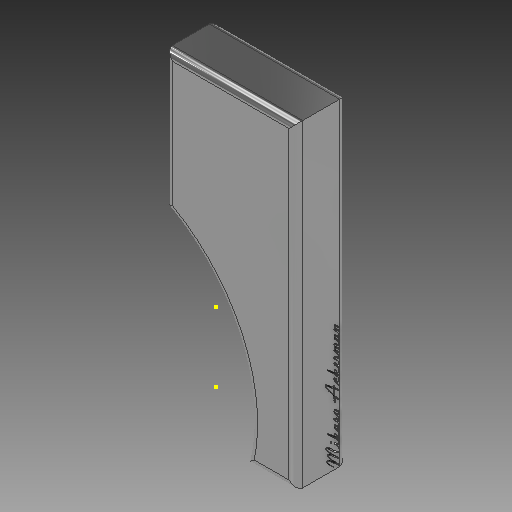
# Autodesk Inventor part: Wire Attachement
Saved by Autodesk Inventor 2021 (Build 250183000, 183)
## iProperties
Created: 2021-05-04
Part Number: Wire Attachement
Material: Generic
Document SubType Name: Modeling
Designer: AHUJA
Density: 1 g/cm^3
Appearance: Default
Author: AHUJA
Autodesk Inventor part; units mm, degrees
ref_plane "YZ Plane" through (0, 0, 0) normal (1, 0, 0) x (0, 1, 0)
ref_plane "XZ Plane" through (0, 0, 0) normal (0, 1, 0) x (-1, 0, 0)
ref_plane "XY Plane" through (0, 0, 0) normal (0, 0, 1) x (1, 0, 0)
sketch "Sketch1" plane through (0, 0, 0) normal (0, 0, 1) x (1, 0, 0)
  line L0 (0, 0) -> (18.946, 0)
  line L1 (18.946, 0) -> (18.946, 46.274)
  line L2 (18.946, 46.274) -> (0, 46.274)
  line L3 (0, 46.274) -> (0, 0)
  line L4 (0, 46.274) -> (0, 26.493)
  line L5 (18.946, 0) -> (11.661, 0)
  arc A0 (11.661, 0) -> (0, 26.493) centre (-11.0706, 5.8074) ccw
  dimension "d0" = 46.274
  dimension "d1" = 18.946
  dimension "d2" = 19.781
  dimension "d3" = 7.285
  constraints: 12 end point, 2 parallel, 2 point on circle, 2 point on line, 1 centre point, 1 horizontal, 1 perpendicular
  measures "d0" distance of L0.end L1.end
  measures "d1" distance of L1.end L2.end
  measures "d2" distance of L2.end L4.end
  measures "d3" distance of L0.end L5.end
extrude "Extrusion1" add sketch "Sketch1" along normal blind 7.366 contours A0 L3 L2 L1 L0
fillet "Fillet1" radius 1 10 edges at (10.403, 15.2591, 7.366) (0, 36.3835, 7.366) (9.473, 46.274, 7.366) (18.946, 23.137, 7.366) (15.3035, 0, 7.366) (18.946, 23.137, 0) (15.3035, 0, 0) (10.403, 15.2591, 0) (0, 36.3835, 0) (9.473, 46.274, 0)
sketch "Sketch2" plane through (11.661, 0, 1) normal (0, -1, 0) x (1, 0, 0)
  point P0 (-11.661, -1)
sketch "Sketch3" plane through (11.661, 0, 1) normal (0, -1, 0) x (1, 0, 0)
  line L0 (1.21, 5.156) -> (6.075, 5.156)
  line L1 (6.075, 5.156) -> (6.075, 0.21)
  line L2 (6.075, 0.21) -> (1.21, 0.21)
  line L3 (1.21, 0.21) -> (1.21, 5.156)
  line L4 (6.285, 6.366) -> (1.2531, 6.366) projected
  line L5 (1.2531, -1) -> (6.285, -1) projected
  line L6 (7.285, 0) -> (7.285, 5.366) projected
  line L7 (0, 0) -> (0, 5.366) projected
  point P0 (-11.661, -1)
  dimension "d7" = 1.21
  dimension "d8" = 1.21
  dimension "d9" = 1.21
  dimension "d10" = 1.21
  constraints: 8 end point, 2 parallel, 1 horizontal, 1 perpendicular
  measures "d7" distance between parallel lines of L4 L0
  measures "d8" distance between parallel lines of L5 L2
  measures "d9" distance between parallel lines of L6 L1
  measures "d10" distance between parallel lines of L7 L3
extrude "Extrusion2" cut sketch "Sketch3" against normal blind 10.16
fillet "Fillet2" radius 0.25 4 edges at (12.871, 5.08, 1.21) (12.871, 5.08, 6.156) (17.736, 5.08, 1.21) (17.736, 5.08, 6.156)
sketch "Sketch4" plane through (11.661, 10.16, 1) normal (0, -1, 0) x (1, 0, 0)
  line L0 (1.61, 3.51) -> (2.41, 3.51)
  line L1 (2.41, 3.51) -> (2.41, 2.41)
  line L2 (2.41, 2.41) -> (1.61, 2.41)
  line L3 (1.61, 2.41) -> (1.61, 3.51)
  line L4 (1.21, 0.46) -> (1.21, 4.906) projected
  line L5 (5.825, 0.21) -> (1.46, 0.21) projected
  line L6 (2.81, 3.51) -> (3.61, 3.51)
  line L7 (3.61, 3.51) -> (3.61, 2.41)
  line L8 (3.61, 2.41) -> (2.81, 2.41)
  line L9 (2.81, 2.41) -> (2.81, 3.51)
  point P0 (-11.661, -1)
  dimension "d14" = 0.4
  dimension "d15" = 0.8
  dimension "d16" = 1.1
  dimension "d17" = 2.2
  dimension "d18" = 0.8
  dimension "d19" = 1.1
  dimension "d20" = 0.4
  dimension "d21" = 2.2
  constraints: 16 end point, 4 parallel, 2 horizontal, 2 perpendicular
  measures "d14" distance between parallel lines of L4 L3
  measures "d15" distance of L0.start L0.end
  measures "d16" distance of L0.end L1.end
  measures "d17" distance between parallel lines of L5 L2
  measures "d18" distance of L6.start L6.end
  measures "d19" distance of L6.end L7.end
  measures "d20" distance between parallel lines of L1 L9
  measures "d21" distance between parallel lines of L5 L8
extrude "Extrusion3" add sketch "Sketch4" along normal blind 10.16
fillet "Fillet3" radius 0.15 8 edges at (15.271, 5.08, 4.51) (15.271, 5.08, 3.41) (14.071, 5.08, 3.41) (14.071, 5.08, 4.51) (14.471, 5.08, 4.51) (14.471, 5.08, 3.41) (13.271, 5.08, 4.51) (13.271, 5.08, 3.41)
sketch "Sketch5" plane through (11.661, 10.16, 1) normal (0, -1, 0) x (1, 0, 0)
  point P0 (-11.661, -1)
sketch "Sketch6" plane through (11.661, 10.16, 1) normal (0, -1, 0) x (1, 0, 0)
  line L0 (3.91, 3.91) -> (5.91, 3.91)
  line L1 (5.91, 3.91) -> (5.91, 2.21)
  line L2 (5.91, 2.21) -> (3.91, 2.21)
  line L3 (3.91, 2.21) -> (3.91, 3.91)
  line L4 (1.46, 5.156) -> (5.825, 5.156) projected
  line L5 (5.825, 0.21) -> (1.46, 0.21) projected
  line L6 (3.61, 2.56) -> (3.61, 3.36) projected
  point P0 (-11.661, -1)
  dimension "d25" = 2
  dimension "d26" = 1.7
  dimension "d28" = 2
  dimension "d29" = 0.3
  constraints: 8 end point, 2 parallel, 1 horizontal, 1 perpendicular
  measures "d25" distance of L0.start L0.end
  measures "d26" distance of L2.end L0.start
  measures "d28" distance between parallel lines of L5 L2
  measures "d29" distance between parallel lines of L6 L3
extrude "Extrusion4" add sketch "Sketch6" along normal blind 10.16
sketch "Sketch7" plane through (11.661, 0, 1) normal (0, -1, 0) x (1, 0, 0)
  line L0 (4.31, 3.51) -> (5.51, 3.51)
  line L1 (5.51, 3.51) -> (5.51, 2.61)
  line L2 (5.51, 2.61) -> (4.31, 2.61)
  line L3 (4.31, 2.61) -> (4.31, 3.51)
  line L4 (5.91, 3.91) -> (3.91, 3.91) projected
  line L5 (3.91, 2.21) -> (5.91, 2.21) projected
  line L6 (5.91, 2.21) -> (5.91, 3.91) projected
  line L7 (3.91, 3.91) -> (3.91, 2.21) projected
  point P0 (-11.661, -1)
  dimension "d32" = 0.4
  dimension "d33" = 0.4
  dimension "d34" = 0.4
  dimension "d35" = 0.4
  constraints: 8 end point, 2 parallel, 1 horizontal, 1 perpendicular
  measures "d32" distance between parallel lines of L4 L0
  measures "d33" distance between parallel lines of L5 L2
  measures "d34" distance between parallel lines of L6 L1
  measures "d35" distance between parallel lines of L3 L7
extrude "Extrusion5" cut sketch "Sketch7" against normal blind 10.16 contours L0 L1 L2 L3
fillet "Fillet4" radius 0.15 4 edges at (17.571, 5.08, 4.91) (17.571, 5.08, 3.21) (15.571, 5.08, 4.91) (15.571, 5.08, 3.21)
sketch "Sketch8" plane through (18.946, 0, 1) normal (1, 0, 0) x (0, 0, -1)
  line L0 (-2.1201, 0.0445) -> (-2.1201, 18.5514) construction
  line L1 (-2.1201, 18.5514) -> (-0.0042, 18.5514) construction
  line L2 (-0.0042, 18.5514) -> (-0.0042, 0.0445) construction
  line L3 (-0.0042, 0.0445) -> (-2.1201, 0.0445) construction
  spline S0 degree 2 poles (-1.0025, 1.9649) (-2.0042, 2.9545) (-2.0042, 3.2314) knots 0 0 0 1 1 1
  spline S1 degree 2 poles (-2.0042, 3.2314) (-2.0042, 3.3473) (-1.8952, 3.3473) knots 0 0 0 1 1 1
  spline S2 degree 2 poles (-1.8952, 3.3473) (-1.7932, 3.3473) (-1.6686, 3.2642) knots 0 0 0 1 1 1
  spline S3 degree 2 poles (-1.6686, 3.2642) (-1.5804, 3.202) (-0.8624, 2.5168) knots 0 0 0 1 1 1
  spline S4 degree 2 poles (-0.8624, 2.5168) (-0.2291, 1.9459) (-0.1184, 1.9459) knots 0 0 0 1 1 1
  spline S5 degree 2 poles (-0.1184, 1.9459) (-0.0804, 1.9459) (-0.0717, 2.0566) (-0.0596, 2.0566) knots 0 0 0 1 2 2 2
  spline S6 degree 2 poles (-0.0596, 2.0566) (-0.0198, 2.0566) (-0.0198, 1.9701) knots 0 0 0 1 1 1
  spline S7 degree 2 poles (-0.0198, 1.9701) (-0.0198, 1.8473) (-0.1357, 1.8473) knots 0 0 0 1 1 1
  spline S8 degree 2 poles (-0.1357, 1.8473) (-0.3502, 1.8473) (-0.9437, 2.3802) knots 0 0 0 1 1 1
  spline S9 degree 2 poles (-0.9437, 2.3802) (-1.153, 2.567) (-1.6755, 3.0878) knots 0 0 0 1 1 1
  spline S10 degree 2 poles (-1.6755, 3.0878) (-1.852, 3.266) (-1.9229, 3.266) knots 0 0 0 1 1 1
  spline S11 degree 2 poles (-1.9229, 3.266) (-1.9506, 3.266) (-1.9506, 3.2383) knots 0 0 0 1 1 1
  spline S12 degree 2 poles (-1.9506, 3.2383) (-1.9506, 3.1397) (-1.5717, 2.6829) knots 0 0 0 1 1 1
  spline S13 degree 2 poles (-1.5717, 2.6829) (-1.2672, 2.3179) (-1.0873, 2.1379) knots 0 0 0 1 1 1
  spline S14 degree 2 poles (-1.0873, 2.1379) (-0.9143, 1.9649) (-0.5994, 1.6829) knots 0 0 0 1 1 1
  spline S15 degree 2 poles (-0.5994, 1.6829) (-0.0302, 1.176) (-0.0302, 1.1604) knots 0 0 0 1 1 1
  spline S16 degree 2 poles (-0.0302, 1.1604) (-0.0302, 1.1397) (-0.0838, 1.0808) (-0.1063, 1.0808) knots 0 0 0 1 2 2 2
  spline S17 degree 2 poles (-0.1063, 1.0808) (-0.1617, 1.0808) (-1.5942, 2.2936) (-1.7084, 2.2936) knots 0 0 0 1 2 2 2
  spline S18 degree 2 poles (-1.7084, 2.2936) (-1.7378, 2.2936) (-1.7378, 2.266) knots 0 0 0 1 1 1
  spline S19 degree 2 poles (-1.7378, 2.266) (-1.7378, 2.1916) (-1.5094, 1.8888) knots 0 0 0 1 1 1
  spline S20 degree 2 poles (-1.5094, 1.8888) (-1.2983, 1.6085) (-0.9783, 1.2729) knots 0 0 0 1 1 1
  line L4 (-0.9783, 1.2729) -> (-0.4056, 0.695)
  line L5 (-0.4056, 0.695) -> (-0.1876, 0.4926)
  spline S21 degree 2 poles (-0.1876, 0.4926) (-0.0042, 0.3231) (-0.0042, 0.3092) knots 0 0 0 1 1 1
  spline S22 degree 2 poles (-0.0042, 0.3092) (-0.0042, 0.2867) (-0.0267, 0.2521) knots 0 0 0 1 1 1
  spline S23 degree 2 poles (-0.0267, 0.2521) (-0.0509, 0.2141) (-0.0734, 0.2141) knots 0 0 0 1 1 1
  spline S24 degree 2 poles (-0.0734, 0.2141) (-0.1201, 0.2141) (-0.5215, 0.5722) knots 0 0 0 1 1 1
  line L6 (-0.5215, 0.5722) -> (-1.2724, 1.24)
  spline S25 degree 2 poles (-1.2724, 1.24) (-1.6945, 1.5999) (-1.7949, 1.5999) knots 0 0 0 1 1 1
  spline S26 degree 2 poles (-1.7949, 1.5999) (-1.8312, 1.5999) (-1.8312, 1.5635) knots 0 0 0 1 1 1
  spline S27 degree 2 poles (-1.8312, 1.5635) (-1.8312, 1.4597) (-1.5665, 1.1345) knots 0 0 0 1 1 1
  spline S28 degree 2 poles (-1.5665, 1.1345) (-1.3693, 0.8905) (-0.8676, 0.439) knots 0 0 0 1 1 1
  spline S29 degree 2 poles (-0.8676, 0.439) (-0.8364, 0.4096) (-0.8364, 0.3923) knots 0 0 0 1 1 1
  spline S30 degree 2 poles (-0.8364, 0.3923) (-0.8364, 0.3611) (-0.8606, 0.3611) knots 0 0 0 1 1 1
  spline S31 degree 2 poles (-0.8606, 0.3611) (-0.897, 0.3611) (-1.1842, 0.6103) knots 0 0 0 1 1 1
  spline S32 degree 2 poles (-1.1842, 0.6103) (-1.3866, 0.7902) (-1.6132, 1.0618) knots 0 0 0 1 1 1
  spline S33 degree 2 poles (-1.6132, 1.0618) (-1.9039, 1.4148) (-1.9039, 1.5722) knots 0 0 0 1 1 1
  spline S34 degree 2 poles (-1.9039, 1.5722) (-1.9039, 1.6777) (-1.788, 1.6777) knots 0 0 0 1 1 1
  spline S35 degree 2 poles (-1.788, 1.6777) (-1.5942, 1.6777) (-0.9662, 1.1639) knots 0 0 0 1 1 1
  spline S36 degree 2 poles (-0.9662, 1.1639) (-1.8018, 2.0411) (-1.8018, 2.266) knots 0 0 0 1 1 1
  spline S37 degree 2 poles (-1.8018, 2.266) (-1.8018, 2.3715) (-1.6928, 2.3715) knots 0 0 0 1 1 1
  spline S38 degree 2 poles (-1.6928, 2.3715) (-1.5215, 2.3715) (-1.0025, 1.9649) knots 0 0 0 1 1 1
  spline S39 degree 2 poles (-0.1167, 2.9459) (-0.0786, 2.9459) (-0.0786, 3.0289) knots 0 0 0 1 1 1
  spline S40 degree 2 poles (-0.0786, 3.0289) (-0.0786, 3.048) (-0.0544, 3.048) knots 0 0 0 1 1 1
  spline S41 degree 2 poles (-0.0544, 3.048) (-0.0267, 3.048) (-0.0267, 2.9528) knots 0 0 0 1 1 1
  spline S42 degree 2 poles (-0.0267, 2.9528) (-0.0267, 2.8455) (-0.1288, 2.8455) knots 0 0 0 1 1 1
  spline S43 degree 2 poles (-0.1288, 2.8455) (-0.2499, 2.8455) (-0.6305, 3.1639) knots 0 0 0 1 1 1
  line L7 (-0.6305, 3.1639) -> (-0.3122, 2.7746)
  spline S44 degree 2 poles (-0.3122, 2.7746) (-0.0302, 2.4286) (-0.0302, 2.2729) knots 0 0 0 1 1 1
  spline S45 degree 2 poles (-0.0302, 2.2729) (-0.0302, 2.2556) (-0.0492, 2.2556) knots 0 0 0 1 1 1
  spline S46 degree 2 poles (-0.0492, 2.2556) (-0.0769, 2.2556) (-0.0821, 2.285) knots 0 0 0 1 1 1
  spline S47 degree 2 poles (-0.0821, 2.285) (-0.0994, 2.3732) (-0.1409, 2.4476) knots 0 0 0 1 1 1
  spline S48 degree 2 poles (-0.1409, 2.4476) (-0.1911, 2.5411) (-0.4298, 2.8421) knots 0 0 0 1 1 1
  line L8 (-0.4298, 2.8421) -> (-0.7949, 3.2781)
  spline S49 degree 2 poles (-0.7949, 3.2781) (-0.8053, 3.3075) (-0.8053, 3.3559) knots 0 0 0 1 1 1
  spline S50 degree 2 poles (-0.8053, 3.3559) (-0.8053, 3.4044) (-0.7499, 3.4044) knots 0 0 0 1 1 1
  spline S51 degree 2 poles (-0.7499, 3.4044) (-0.6893, 3.4044) (-0.1634, 2.9459) (-0.1167, 2.9459) knots 0 0 0 1 2 2 2
  spline S52 degree 2 poles (-1.1046, 3.5757) (-1.1046, 3.5064) (-1.1738, 3.5064) knots 0 0 0 1 1 1
  spline S53 degree 2 poles (-1.1738, 3.5064) (-1.2326, 3.5064) (-1.2793, 3.5757) knots 0 0 0 1 1 1
  spline S54 degree 2 poles (-1.2793, 3.5757) (-1.3226, 3.6397) (-1.3226, 3.702) knots 0 0 0 1 1 1
  spline S55 degree 2 poles (-1.3226, 3.702) (-1.3226, 3.7763) (-1.2413, 3.7763) knots 0 0 0 1 1 1
  spline S56 degree 2 poles (-1.2413, 3.7763) (-1.1824, 3.7763) (-1.1409, 3.702) knots 0 0 0 1 1 1
  spline S57 degree 2 poles (-1.1409, 3.702) (-1.1046, 3.6379) (-1.1046, 3.5757) knots 0 0 0 1 1 1
  line L9 (-0.6893, 3.977) -> (-0.3676, 3.5947)
  line L10 (-0.3676, 3.5947) -> (-0.1617, 3.3317)
  spline S58 degree 2 poles (-0.1617, 3.3317) (-0.0302, 3.1449) (-0.0302, 3.0255) knots 0 0 0 1 1 1
  spline S59 degree 2 poles (-0.0302, 3.0255) (-0.0302, 3.0082) (-0.0492, 3.0082) knots 0 0 0 1 1 1
  spline S60 degree 2 poles (-0.0492, 3.0082) (-0.0752, 3.0082) (-0.0821, 3.0376) knots 0 0 0 1 1 1
  spline S61 degree 2 poles (-0.0821, 3.0376) (-0.1271, 3.2244) (-0.3935, 3.5462) knots 0 0 0 1 1 1
  line L11 (-0.3935, 3.5462) -> (-0.7326, 3.9528)
  spline S62 degree 2 poles (-0.7326, 3.9528) (-0.8502, 4.093) (-1.1963, 4.4044) knots 0 0 0 1 1 1
  line L12 (-1.1963, 4.4044) -> (-1.653, 4.804)
  spline S63 degree 2 poles (-1.653, 4.804) (-1.7655, 4.8992) (-1.7655, 4.9372) knots 0 0 0 1 1 1
  spline S64 degree 2 poles (-1.7655, 4.9372) (-1.7655, 4.9874) (-1.7153, 4.9874) knots 0 0 0 1 1 1
  spline S65 degree 2 poles (-1.7153, 4.9874) (-1.653, 4.9874) (-1.5008, 4.8646) knots 0 0 0 1 1 1
  line L13 (-1.5008, 4.8646) -> (-1.3001, 4.6881)
  line L14 (-1.3001, 4.6881) -> (-0.6444, 4.1189)
  spline S66 degree 2 poles (-0.6444, 4.1189) (-0.7949, 4.3282) (-0.7949, 4.4269) knots 0 0 0 1 1 1
  spline S67 degree 2 poles (-0.7949, 4.4269) (-0.7949, 4.5428) (-0.6807, 4.5428) knots 0 0 0 1 1 1
  spline S68 degree 2 poles (-0.6807, 4.5428) (-0.5527, 4.5428) (-0.461, 4.3179) knots 0 0 0 1 1 1
  spline S69 degree 2 poles (-0.461, 4.3179) (-0.3866, 4.1345) (-0.3849, 3.977) knots 0 0 0 1 1 1
  spline S70 degree 2 poles (-0.3849, 3.977) (-0.2637, 4.0272) (-0.1098, 4.1085) knots 0 0 0 1 1 1
  spline S71 degree 2 poles (-0.1098, 4.1085) (-0.0769, 4.1362) (-0.0769, 4.1968) knots 0 0 0 1 1 1
  spline S72 degree 2 poles (-0.0769, 4.1968) (-0.0769, 4.2175) (-0.0544, 4.2175) knots 0 0 0 1 1 1
  spline S73 degree 2 poles (-0.0544, 4.2175) (-0.0233, 4.2175) (-0.0233, 4.1068) knots 0 0 0 1 1 1
  spline S74 degree 2 poles (-0.0233, 4.1068) (-0.0233, 4.0514) (-0.0509, 4.0134) knots 0 0 0 1 1 1
  spline S75 degree 2 poles (-0.0509, 4.0134) (-0.0752, 3.9788) (-0.3329, 3.8577) knots 0 0 0 1 1 1
  line L15 (-0.3329, 3.8577) -> (-0.1617, 3.7141)
  spline S76 degree 2 poles (-0.1617, 3.7141) (-0.0215, 3.5947) (-0.0215, 3.5705) knots 0 0 0 1 1 1
  spline S77 degree 2 poles (-0.0215, 3.5705) (-0.0215, 3.5099) (-0.0925, 3.5099) knots 0 0 0 1 1 1
  spline S78 degree 2 poles (-0.0925, 3.5099) (-0.134, 3.5099) (-0.4056, 3.7348) knots 0 0 0 1 1 1
  line L16 (-0.4056, 3.7348) -> (-0.6893, 3.977)
  spline S79 degree 2 poles (-0.4177, 3.9338) (-0.4454, 4.1466) (-0.6253, 4.4234) (-0.6893, 4.4234) knots 0 0 0 1 2 2 2
  spline S80 degree 2 poles (-0.6893, 4.4234) (-0.7222, 4.4234) (-0.7222, 4.3819) knots 0 0 0 1 1 1
  spline S81 degree 2 poles (-0.7222, 4.3819) (-0.7222, 4.2262) (-0.4177, 3.9338) knots 0 0 0 1 1 1
  spline S82 degree 2 poles (-0.3312, 4.721) (-0.0302, 4.3386) (-0.0302, 4.195) knots 0 0 0 1 1 1
  spline S83 degree 2 poles (-0.0302, 4.195) (-0.0302, 4.1777) (-0.0492, 4.1777) knots 0 0 0 1 1 1
  spline S84 degree 2 poles (-0.0492, 4.1777) (-0.0769, 4.1777) (-0.0821, 4.2123) knots 0 0 0 1 1 1
  spline S85 degree 2 poles (-0.0821, 4.2123) (-0.1028, 4.3455) (-0.2897, 4.5843) knots 0 0 0 1 1 1
  line L17 (-0.2897, 4.5843) -> (-0.4333, 4.7677)
  line L18 (-0.4333, 4.7677) -> (-0.6686, 5.0635)
  spline S86 degree 2 poles (-0.6686, 5.0635) (-0.8087, 5.266) (-0.8087, 5.4113) knots 0 0 0 1 1 1
  spline S87 degree 2 poles (-0.8087, 5.4113) (-0.8087, 5.5186) (-0.7015, 5.5307) knots 0 0 0 1 1 1
  spline S88 degree 2 poles (-0.7015, 5.5307) (-0.7551, 5.586) (-0.7551, 5.6085) knots 0 0 0 1 1 1
  spline S89 degree 2 poles (-0.7551, 5.6085) (-0.7551, 5.6552) (-0.7153, 5.6552) knots 0 0 0 1 1 1
  spline S90 degree 2 poles (-0.7153, 5.6552) (-0.6651, 5.6552) (-0.1547, 5.2175) (-0.1115, 5.2175) knots 0 0 0 1 2 2 2
  spline S91 degree 2 poles (-0.1115, 5.2175) (-0.0821, 5.2175) (-0.0786, 5.3092) (-0.0561, 5.3092) knots 0 0 0 1 2 2 2
  spline S92 degree 2 poles (-0.0561, 5.3092) (-0.0267, 5.3092) (-0.0267, 5.2141) knots 0 0 0 1 1 1
  spline S93 degree 2 poles (-0.0267, 5.2141) (-0.0267, 5.1189) (-0.1115, 5.1189) knots 0 0 0 1 1 1
  spline S94 degree 2 poles (-0.1115, 5.1189) (-0.179, 5.1189) (-0.3018, 5.195) knots 0 0 0 1 1 1
  line L19 (-0.3018, 5.195) -> (-0.1513, 5.0186)
  spline S95 degree 2 poles (-0.1513, 5.0186) (-0.0544, 4.8888) (-0.0544, 4.8109) knots 0 0 0 1 1 1
  spline S96 degree 2 poles (-0.0544, 4.8109) (-0.0544, 4.6881) (-0.179, 4.6881) knots 0 0 0 1 1 1
  spline S97 degree 2 poles (-0.179, 4.6881) (-0.2482, 4.6881) (-0.3312, 4.721) knots 0 0 0 1 1 1
  spline S98 degree 2 poles (-0.7499, 5.4303) (-0.7499, 5.3455) (-0.2464, 4.8179) (-0.1617, 4.8179) knots 0 0 0 1 2 2 2
  spline S99 degree 2 poles (-0.1617, 4.8179) (-0.1236, 4.8179) (-0.1236, 4.8542) knots 0 0 0 1 1 1
  spline S100 degree 2 poles (-0.1236, 4.8542) (-0.1236, 4.9372) (-0.6167, 5.4718) (-0.7032, 5.4718) knots 0 0 0 1 2 2 2
  spline S101 degree 2 poles (-0.7032, 5.4718) (-0.7499, 5.4718) (-0.7499, 5.4303) knots 0 0 0 1 1 1
  spline S102 degree 2 poles (-0.2741, 5.7383) (-0.0302, 5.4407) (-0.0302, 5.2867) knots 0 0 0 1 1 1
  spline S103 degree 2 poles (-0.0302, 5.2867) (-0.0302, 5.2694) (-0.0475, 5.2694) knots 0 0 0 1 1 1
  spline S104 degree 2 poles (-0.0475, 5.2694) (-0.0752, 5.2694) (-0.0821, 5.2988) knots 0 0 0 1 1 1
  spline S105 degree 2 poles (-0.0821, 5.2988) (-0.0942, 5.3507) (-0.1392, 5.4615) knots 0 0 0 1 1 1
  spline S106 degree 2 poles (-0.1392, 5.4615) (-0.1945, 5.5635) (-0.544, 5.984) knots 0 0 0 1 1 1
  spline S107 degree 2 poles (-0.544, 5.984) (-0.8745, 6.3819) (-0.8745, 6.3923) knots 0 0 0 1 1 1
  spline S108 degree 2 poles (-0.8745, 6.3923) (-0.8745, 6.4251) (-0.8174, 6.4891) (-0.7845, 6.4891) knots 0 0 0 1 2 2 2
  spline S109 degree 2 poles (-0.7845, 6.4891) (-0.6807, 6.4891) (-0.4177, 6.3265) knots 0 0 0 1 1 1
  spline S110 degree 2 poles (-0.4177, 6.3265) (-0.1911, 6.1847) (-0.0786, 6.0791) knots 0 0 0 1 1 1
  spline S111 degree 2 poles (-0.0786, 6.0791) (-0.0786, 6.1414) (-0.0561, 6.1414) knots 0 0 0 1 1 1
  spline S112 degree 2 poles (-0.0561, 6.1414) (-0.0267, 6.1414) (-0.0267, 6.0808) knots 0 0 0 1 1 1
  spline S113 degree 2 poles (-0.0267, 6.0808) (-0.0267, 6.0653) (-0.0371, 6.0047) (-0.0371, 5.9874) knots 0 0 0 1 2 2 2
  spline S114 degree 2 poles (-0.0371, 5.9874) (-0.0371, 5.977) (-0.0284, 5.9303) (-0.0284, 5.9199) knots 0 0 0 1 2 2 2
  spline S115 degree 2 poles (-0.0284, 5.9199) (-0.0284, 5.7383) (-0.2741, 5.7383) knots 0 0 0 1 1 1
  spline S116 degree 2 poles (-0.1478, 5.9649) (-0.2309, 6.0653) (-0.435, 6.1847) knots 0 0 0 1 1 1
  spline S117 degree 2 poles (-0.435, 6.1847) (-0.6236, 6.2954) (-0.7689, 6.3404) knots 0 0 0 1 1 1
  line L20 (-0.7689, 6.3404) -> (-0.3537, 5.83)
  spline S118 degree 2 poles (-0.3537, 5.83) (-0.3451, 5.8819) (-0.2707, 5.9182) knots 0 0 0 1 1 1
  line L21 (-0.2707, 5.9182) -> (-0.1478, 5.9649)
  line L22 (-0.1046, 5.9251) -> (-0.2188, 5.8853)
  spline S119 degree 2 poles (-0.2188, 5.8853) (-0.3018, 5.8525) (-0.3018, 5.8231) knots 0 0 0 1 1 1
  spline S120 degree 2 poles (-0.3018, 5.8231) (-0.3018, 5.7919) (-0.2534, 5.7919) knots 0 0 0 1 1 1
  spline S121 degree 2 poles (-0.2534, 5.7919) (-0.2032, 5.7919) (-0.1513, 5.8196) knots 0 0 0 1 1 1
  spline S122 degree 2 poles (-0.1513, 5.8196) (-0.0925, 5.8525) (-0.0925, 5.8975) knots 0 0 0 1 1 1
  spline S123 degree 2 poles (-0.0925, 5.8975) (-0.0925, 5.9148) (-0.1046, 5.9251) knots 0 0 0 1 1 1
  spline S124 degree 2 poles (-0.3312, 6.6449) (-0.0302, 6.2625) (-0.0302, 6.1189) knots 0 0 0 1 1 1
  spline S125 degree 2 poles (-0.0302, 6.1189) (-0.0302, 6.1016) (-0.0492, 6.1016) knots 0 0 0 1 1 1
  spline S126 degree 2 poles (-0.0492, 6.1016) (-0.0769, 6.1016) (-0.0821, 6.1362) knots 0 0 0 1 1 1
  spline S127 degree 2 poles (-0.0821, 6.1362) (-0.1028, 6.2694) (-0.2897, 6.5082) knots 0 0 0 1 1 1
  line L23 (-0.2897, 6.5082) -> (-0.4333, 6.6916)
  line L24 (-0.4333, 6.6916) -> (-0.6686, 6.9874)
  spline S128 degree 2 poles (-0.6686, 6.9874) (-0.8087, 7.1898) (-0.8087, 7.3352) knots 0 0 0 1 1 1
  spline S129 degree 2 poles (-0.8087, 7.3352) (-0.8087, 7.4424) (-0.7015, 7.4545) knots 0 0 0 1 1 1
  spline S130 degree 2 poles (-0.7015, 7.4545) (-0.7551, 7.5099) (-0.7551, 7.5324) knots 0 0 0 1 1 1
  spline S131 degree 2 poles (-0.7551, 7.5324) (-0.7551, 7.5791) (-0.7153, 7.5791) knots 0 0 0 1 1 1
  spline S132 degree 2 poles (-0.7153, 7.5791) (-0.6651, 7.5791) (-0.1547, 7.1414) (-0.1115, 7.1414) knots 0 0 0 1 2 2 2
  spline S133 degree 2 poles (-0.1115, 7.1414) (-0.0821, 7.1414) (-0.0786, 7.2331) (-0.0561, 7.2331) knots 0 0 0 1 2 2 2
  spline S134 degree 2 poles (-0.0561, 7.2331) (-0.0267, 7.2331) (-0.0267, 7.1379) knots 0 0 0 1 1 1
  spline S135 degree 2 poles (-0.0267, 7.1379) (-0.0267, 7.0428) (-0.1115, 7.0428) knots 0 0 0 1 1 1
  spline S136 degree 2 poles (-0.1115, 7.0428) (-0.179, 7.0428) (-0.3018, 7.1189) knots 0 0 0 1 1 1
  line L25 (-0.3018, 7.1189) -> (-0.1513, 6.9424)
  spline S137 degree 2 poles (-0.1513, 6.9424) (-0.0544, 6.8127) (-0.0544, 6.7348) knots 0 0 0 1 1 1
  spline S138 degree 2 poles (-0.0544, 6.7348) (-0.0544, 6.612) (-0.179, 6.612) knots 0 0 0 1 1 1
  spline S139 degree 2 poles (-0.179, 6.612) (-0.2482, 6.612) (-0.3312, 6.6449) knots 0 0 0 1 1 1
  spline S140 degree 2 poles (-0.7499, 7.3542) (-0.7499, 7.2694) (-0.2464, 6.7417) (-0.1617, 6.7417) knots 0 0 0 1 2 2 2
  spline S141 degree 2 poles (-0.1617, 6.7417) (-0.1236, 6.7417) (-0.1236, 6.7781) knots 0 0 0 1 1 1
  spline S142 degree 2 poles (-0.1236, 6.7781) (-0.1236, 6.8611) (-0.6167, 7.3957) (-0.7032, 7.3957) knots 0 0 0 1 2 2 2
  spline S143 degree 2 poles (-0.7032, 7.3957) (-0.7499, 7.3957) (-0.7499, 7.3542) knots 0 0 0 1 1 1
  line L26 (-0.8537, 10.4199) -> (-0.8537, 10.5497)
  spline S144 degree 2 poles (-0.8537, 10.5497) (-0.8433, 10.6449) (-0.7949, 10.6449) knots 0 0 0 1 1 1
  spline S145 degree 2 poles (-0.7949, 10.6449) (-0.7637, 10.6449) (-0.7637, 10.5757) knots 0 0 0 1 1 1
  line L27 (-0.7637, 10.5757) -> (-0.7689, 10.484)
  line L28 (-0.7689, 10.484) -> (-0.7672, 10.349)
  line L29 (-0.7672, 10.349) -> (-0.3987, 10.0584)
  spline S146 degree 2 poles (-0.3987, 10.0584) (-0.0302, 9.7625) (-0.0302, 9.7314) knots 0 0 0 1 1 1
  spline S147 degree 2 poles (-0.0302, 9.7314) (-0.0302, 9.7037) (-0.0717, 9.6812) knots 0 0 0 1 1 1
  spline S148 degree 2 poles (-0.0717, 9.6812) (-0.1063, 9.6587) (-0.1357, 9.6587) knots 0 0 0 1 1 1
  spline S149 degree 2 poles (-0.1357, 9.6587) (-0.1807, 9.6587) (-0.7672, 10.1449) knots 0 0 0 1 1 1
  line L30 (-0.7672, 10.1449) -> (-0.7672, 10.0341)
  spline S150 degree 2 poles (-0.7672, 10.0341) (-0.7655, 9.8006) (-0.743, 9.3404) knots 0 0 0 1 1 1
  line L31 (-0.743, 9.3404) -> (-0.3295, 8.8594)
  line L32 (-0.3295, 8.8594) -> (-0.1617, 8.6708)
  spline S151 degree 2 poles (-0.1617, 8.6708) (-0.0302, 8.5203) (-0.0302, 8.4874) knots 0 0 0 1 1 1
  spline S152 degree 2 poles (-0.0302, 8.4874) (-0.0302, 8.4476) (-0.0717, 8.4476) knots 0 0 0 1 1 1
  spline S153 degree 2 poles (-0.0717, 8.4476) (-0.1236, 8.4476) (-0.4679, 8.8594) knots 0 0 0 1 1 1
  line L33 (-0.4679, 8.8594) -> (-0.7395, 9.1864)
  spline S154 degree 2 poles (-0.7395, 9.1864) (-0.7084, 8.5324) (-0.672, 8.5116) knots 0 0 0 1 1 1
  line L34 (-0.672, 8.5116) -> (-0.6703, 8.5116)
  spline S155 degree 2 poles (-0.6703, 8.5116) (-0.6426, 8.5116) (-0.6426, 8.7158) knots 0 0 0 1 1 1
  line L35 (-0.6426, 8.7158) -> (-0.6461, 8.9061)
  spline S156 degree 2 poles (-0.6461, 8.9061) (-0.6461, 8.9442) (-0.6288, 8.9442) knots 0 0 0 1 1 1
  spline S157 degree 2 poles (-0.6288, 8.9442) (-0.589, 8.9442) (-0.589, 8.6327) knots 0 0 0 1 1 1
  spline S158 degree 2 poles (-0.589, 8.6327) (-0.589, 8.368) (-0.6565, 8.368) knots 0 0 0 1 1 1
  spline S159 degree 2 poles (-0.6565, 8.368) (-0.743, 8.368) (-0.7759, 8.5255) knots 0 0 0 1 1 1
  spline S160 degree 2 poles (-0.7759, 8.5255) (-0.7845, 8.5687) (-0.7966, 8.7452) knots 0 0 0 1 1 1
  line L36 (-0.7966, 8.7452) -> (-0.8329, 9.3006)
  spline S161 degree 2 poles (-0.8329, 9.3006) (-1.1115, 9.6379) (-1.5561, 10.2642) knots 0 0 0 1 1 1
  spline S162 degree 2 poles (-1.5561, 10.2642) (-2.1201, 11.0618) (-2.1201, 11.2158) knots 0 0 0 1 1 1
  spline S163 degree 2 poles (-2.1201, 11.2158) (-2.1201, 11.2936) (-2.0198, 11.2936) knots 0 0 0 1 1 1
  spline S164 degree 2 poles (-2.0198, 11.2936) (-1.935, 11.2936) (-1.6859, 11.093) knots 0 0 0 1 1 1
  line L37 (-1.6859, 11.093) -> (-0.8537, 10.4199)
  line L38 (-0.8537, 10.2158) -> (-1.6651, 10.8836)
  line L39 (-1.6651, 10.8836) -> (-1.8174, 11.0082)
  spline S165 degree 2 poles (-1.8174, 11.0082) (-1.9177, 11.0878) (-1.9731, 11.1137) knots 0 0 0 1 1 1
  line L40 (-1.9731, 11.1137) -> (-1.9783, 11.1154)
  spline S166 degree 2 poles (-1.9783, 11.1154) (-1.9938, 11.1154) (-1.9938, 11.1016) knots 0 0 0 1 1 1
  spline S167 degree 2 poles (-1.9938, 11.1016) (-1.9938, 11.0341) (-1.4229, 10.2521) knots 0 0 0 1 1 1
  line L41 (-1.4229, 10.2521) -> (-0.8399, 9.4684)
  line L42 (-0.8399, 9.4684) -> (-0.8537, 10.2158)
  line L43 (-0.4281, 10.8092) -> (-0.1945, 10.5116)
  spline S168 degree 2 poles (-0.1945, 10.5116) (-0.0302, 10.2798) (-0.0302, 10.1587) knots 0 0 0 1 1 1
  spline S169 degree 2 poles (-0.0302, 10.1587) (-0.0302, 10.1414) (-0.0475, 10.1414) knots 0 0 0 1 1 1
  spline S170 degree 2 poles (-0.0475, 10.1414) (-0.0752, 10.1414) (-0.0821, 10.176) knots 0 0 0 1 1 1
  spline S171 degree 2 poles (-0.0821, 10.176) (-0.108, 10.3092) (-0.2793, 10.5359) knots 0 0 0 1 1 1
  line L44 (-0.2793, 10.5359) -> (-0.5959, 10.9321)
  spline S172 degree 2 poles (-0.5959, 10.9321) (-0.8624, 11.2573) (-0.8624, 11.4321) knots 0 0 0 1 1 1
  spline S173 degree 2 poles (-0.8624, 11.4321) (-0.8624, 11.5255) (-0.7914, 11.5255) knots 0 0 0 1 1 1
  spline S174 degree 2 poles (-0.7914, 11.5255) (-0.7914, 11.5566) (-0.7637, 11.5566) knots 0 0 0 1 1 1
  spline S175 degree 2 poles (-0.7637, 11.5566) (-0.7395, 11.5566) (-0.7378, 11.522) knots 0 0 0 1 1 1
  spline S176 degree 2 poles (-0.7378, 11.522) (-0.6357, 11.4926) (-0.5354, 11.4148) knots 0 0 0 1 1 1
  spline S177 degree 2 poles (-0.5354, 11.4148) (-0.416, 11.3196) (-0.416, 11.2331) knots 0 0 0 1 1 1
  spline S178 degree 2 poles (-0.416, 11.2331) (-0.416, 11.1812) (-0.4627, 11.1812) knots 0 0 0 1 1 1
  spline S179 degree 2 poles (-0.4627, 11.1812) (-0.5302, 11.1812) (-0.6374, 11.2919) knots 0 0 0 1 1 1
  spline S180 degree 2 poles (-0.6374, 11.2919) (-0.7326, 11.3905) (-0.7655, 11.4684) knots 0 0 0 1 1 1
  line L45 (-0.7655, 11.4684) -> (-0.781, 11.4718)
  spline S181 degree 2 poles (-0.781, 11.4718) (-0.8018, 11.4718) (-0.8018, 11.4511) knots 0 0 0 1 1 1
  spline S182 degree 2 poles (-0.8018, 11.4511) (-0.8018, 11.3594) (-0.2914, 10.8629) (-0.1893, 10.8629) knots 0 0 0 1 2 2 2
  spline S183 degree 2 poles (-0.1893, 10.8629) (-0.1253, 10.8629) (-0.1011, 10.9182) knots 0 0 0 1 1 1
  spline S184 degree 2 poles (-0.1011, 10.9182) (-0.0873, 10.9459) (-0.0804, 11.0203) knots 0 0 0 1 1 1
  spline S185 degree 2 poles (-0.0804, 11.0203) (-0.0752, 11.0757) (-0.0561, 11.0757) knots 0 0 0 1 1 1
  spline S186 degree 2 poles (-0.0561, 11.0757) (-0.0267, 11.0757) (-0.0267, 10.9753) knots 0 0 0 1 1 1
  spline S187 degree 2 poles (-0.0267, 10.9753) (-0.0267, 10.7521) (-0.2291, 10.7521) knots 0 0 0 1 1 1
  spline S188 degree 2 poles (-0.2291, 10.7521) (-0.3053, 10.7521) (-0.4281, 10.8092) knots 0 0 0 1 1 1
  spline S189 degree 2 poles (-0.7015, 11.4459) (-0.6824, 11.4044) (-0.608, 11.3282) knots 0 0 0 1 1 1
  spline S190 degree 2 poles (-0.608, 11.3282) (-0.5284, 11.2469) (-0.4973, 11.2469) knots 0 0 0 1 1 1
  line L46 (-0.4973, 11.2469) -> (-0.4852, 11.259)
  spline S191 degree 2 poles (-0.4852, 11.259) (-0.4852, 11.2971) (-0.5734, 11.3663) knots 0 0 0 1 1 1
  spline S192 degree 2 poles (-0.5734, 11.3663) (-0.6496, 11.4234) (-0.7015, 11.4459) knots 0 0 0 1 1 1
  line L47 (-0.6893, 12.0047) -> (-0.3676, 11.6224)
  line L48 (-0.3676, 11.6224) -> (-0.1617, 11.3594)
  spline S193 degree 2 poles (-0.1617, 11.3594) (-0.0302, 11.1725) (-0.0302, 11.0532) knots 0 0 0 1 1 1
  spline S194 degree 2 poles (-0.0302, 11.0532) (-0.0302, 11.0359) (-0.0492, 11.0359) knots 0 0 0 1 1 1
  spline S195 degree 2 poles (-0.0492, 11.0359) (-0.0752, 11.0359) (-0.0821, 11.0653) knots 0 0 0 1 1 1
  spline S196 degree 2 poles (-0.0821, 11.0653) (-0.1271, 11.2521) (-0.3935, 11.5739) knots 0 0 0 1 1 1
  line L49 (-0.3935, 11.5739) -> (-0.7326, 11.9805)
  spline S197 degree 2 poles (-0.7326, 11.9805) (-0.8502, 12.1206) (-1.1963, 12.4321) knots 0 0 0 1 1 1
  line L50 (-1.1963, 12.4321) -> (-1.653, 12.8317)
  spline S198 degree 2 poles (-1.653, 12.8317) (-1.7655, 12.9269) (-1.7655, 12.9649) knots 0 0 0 1 1 1
  spline S199 degree 2 poles (-1.7655, 12.9649) (-1.7655, 13.0151) (-1.7153, 13.0151) knots 0 0 0 1 1 1
  spline S200 degree 2 poles (-1.7153, 13.0151) (-1.653, 13.0151) (-1.5008, 12.8923) knots 0 0 0 1 1 1
  line L51 (-1.5008, 12.8923) -> (-1.3001, 12.7158)
  line L52 (-1.3001, 12.7158) -> (-0.6444, 12.1466)
  spline S201 degree 2 poles (-0.6444, 12.1466) (-0.7949, 12.3559) (-0.7949, 12.4545) knots 0 0 0 1 1 1
  spline S202 degree 2 poles (-0.7949, 12.4545) (-0.7949, 12.5705) (-0.6807, 12.5705) knots 0 0 0 1 1 1
  spline S203 degree 2 poles (-0.6807, 12.5705) (-0.5527, 12.5705) (-0.461, 12.3455) knots 0 0 0 1 1 1
  spline S204 degree 2 poles (-0.461, 12.3455) (-0.3866, 12.1622) (-0.3849, 12.0047) knots 0 0 0 1 1 1
  spline S205 degree 2 poles (-0.3849, 12.0047) (-0.2637, 12.0549) (-0.1098, 12.1362) knots 0 0 0 1 1 1
  spline S206 degree 2 poles (-0.1098, 12.1362) (-0.0769, 12.1639) (-0.0769, 12.2244) knots 0 0 0 1 1 1
  spline S207 degree 2 poles (-0.0769, 12.2244) (-0.0769, 12.2452) (-0.0544, 12.2452) knots 0 0 0 1 1 1
  spline S208 degree 2 poles (-0.0544, 12.2452) (-0.0233, 12.2452) (-0.0233, 12.1345) knots 0 0 0 1 1 1
  spline S209 degree 2 poles (-0.0233, 12.1345) (-0.0233, 12.0791) (-0.0509, 12.0411) knots 0 0 0 1 1 1
  spline S210 degree 2 poles (-0.0509, 12.0411) (-0.0752, 12.0064) (-0.3329, 11.8853) knots 0 0 0 1 1 1
  line L53 (-0.3329, 11.8853) -> (-0.1617, 11.7417)
  spline S211 degree 2 poles (-0.1617, 11.7417) (-0.0215, 11.6224) (-0.0215, 11.5981) knots 0 0 0 1 1 1
  spline S212 degree 2 poles (-0.0215, 11.5981) (-0.0215, 11.5376) (-0.0925, 11.5376) knots 0 0 0 1 1 1
  spline S213 degree 2 poles (-0.0925, 11.5376) (-0.134, 11.5376) (-0.4056, 11.7625) knots 0 0 0 1 1 1
  line L54 (-0.4056, 11.7625) -> (-0.6893, 12.0047)
  spline S214 degree 2 poles (-0.4177, 11.9615) (-0.4454, 12.1743) (-0.6253, 12.4511) (-0.6893, 12.4511) knots 0 0 0 1 2 2 2
  spline S215 degree 2 poles (-0.6893, 12.4511) (-0.7222, 12.4511) (-0.7222, 12.4096) knots 0 0 0 1 1 1
  spline S216 degree 2 poles (-0.7222, 12.4096) (-0.7222, 12.2539) (-0.4177, 11.9615) knots 0 0 0 1 1 1
  spline S217 degree 2 poles (-0.2603, 12.7556) (-0.243, 12.6847) (-0.1288, 12.4874) knots 0 0 0 1 1 1
  spline S218 degree 2 poles (-0.1288, 12.4874) (-0.0302, 12.3127) (-0.0302, 12.2227) knots 0 0 0 1 1 1
  spline S219 degree 2 poles (-0.0302, 12.2227) (-0.0302, 12.2054) (-0.0492, 12.2054) knots 0 0 0 1 1 1
  spline S220 degree 2 poles (-0.0492, 12.2054) (-0.0769, 12.2054) (-0.0821, 12.2417) knots 0 0 0 1 1 1
  spline S221 degree 2 poles (-0.0821, 12.2417) (-0.0959, 12.33) (-0.1876, 12.4874) knots 0 0 0 1 1 1
  spline S222 degree 2 poles (-0.1876, 12.4874) (-0.2862, 12.6622) (-0.3122, 12.7729) knots 0 0 0 1 1 1
  spline S223 degree 2 poles (-0.3122, 12.7729) (-0.4714, 12.8386) (-0.6461, 13.0445) knots 0 0 0 1 1 1
  spline S224 degree 2 poles (-0.6461, 13.0445) (-0.8329, 13.2625) (-0.8329, 13.4165) knots 0 0 0 1 1 1
  spline S225 degree 2 poles (-0.8329, 13.4165) (-0.8329, 13.5307) (-0.7361, 13.5307) knots 0 0 0 1 1 1
  spline S226 degree 2 poles (-0.7361, 13.5307) (-0.608, 13.5307) (-0.4575, 13.2885) knots 0 0 0 1 1 1
  spline S227 degree 2 poles (-0.4575, 13.2885) (-0.3468, 13.112) (-0.2828, 12.9269) knots 0 0 0 1 1 1
  spline S228 degree 2 poles (-0.2828, 12.9269) (-0.2378, 12.9061) (-0.1893, 12.9061) knots 0 0 0 1 1 1
  spline S229 degree 2 poles (-0.1893, 12.9061) (-0.115, 12.9061) (-0.0925, 12.958) knots 0 0 0 1 1 1
  spline S230 degree 2 poles (-0.0925, 12.958) (-0.0838, 12.984) (-0.0804, 13.0549) knots 0 0 0 1 1 1
  spline S231 degree 2 poles (-0.0804, 13.0549) (-0.0786, 13.1068) (-0.0544, 13.1068) knots 0 0 0 1 1 1
  spline S232 degree 2 poles (-0.0544, 13.1068) (-0.0181, 13.1068) (-0.0181, 12.9303) knots 0 0 0 1 1 1
  spline S233 degree 2 poles (-0.0181, 12.9303) (-0.0181, 12.7452) (-0.179, 12.7452) knots 0 0 0 1 1 1
  spline S234 degree 2 poles (-0.179, 12.7452) (-0.2153, 12.7452) (-0.2603, 12.7556) knots 0 0 0 1 1 1
  spline S235 degree 2 poles (-0.3416, 12.9424) (-0.4056, 13.0739) (-0.5163, 13.221) knots 0 0 0 1 1 1
  spline S236 degree 2 poles (-0.5163, 13.221) (-0.6599, 13.4148) (-0.7447, 13.4148) knots 0 0 0 1 1 1
  spline S237 degree 2 poles (-0.7447, 13.4148) (-0.7793, 13.4148) (-0.7793, 13.3836) knots 0 0 0 1 1 1
  spline S238 degree 2 poles (-0.7793, 13.3836) (-0.7793, 13.2902) (-0.608, 13.131) knots 0 0 0 1 1 1
  spline S239 degree 2 poles (-0.608, 13.131) (-0.4506, 12.9874) (-0.3416, 12.9424) knots 0 0 0 1 1 1
  spline S240 degree 2 poles (-0.6617, 13.8888) (-0.7084, 13.8819) (-0.7188, 13.8819) knots 0 0 0 1 1 1
  spline S241 degree 2 poles (-0.7188, 13.8819) (-0.7568, 13.8819) (-0.9212, 14.0653) (-0.9212, 14.0999) knots 0 0 0 1 2 2 2
  spline S242 degree 2 poles (-0.9212, 14.0999) (-0.9212, 14.1327) (-0.8918, 14.1327) knots 0 0 0 1 1 1
  spline S243 degree 2 poles (-0.8918, 14.1327) (-0.8658, 14.1327) (-0.8053, 14.0964) knots 0 0 0 1 1 1
  spline S244 degree 2 poles (-0.8053, 14.0964) (-0.8053, 14.259) (-0.6772, 14.259) knots 0 0 0 1 1 1
  spline S245 degree 2 poles (-0.6772, 14.259) (-0.5769, 14.259) (-0.134, 13.8438) (-0.1063, 13.8438) knots 0 0 0 1 2 2 2
  spline S246 degree 2 poles (-0.1063, 13.8438) (-0.0821, 13.8438) (-0.0786, 13.8715) knots 0 0 0 1 1 1
  line L55 (-0.0786, 13.8715) -> (-0.0804, 13.9182)
  spline S247 degree 2 poles (-0.0804, 13.9182) (-0.0804, 13.9372) (-0.0561, 13.9372) knots 0 0 0 1 1 1
  spline S248 degree 2 poles (-0.0561, 13.9372) (-0.0267, 13.9372) (-0.0267, 13.8542) knots 0 0 0 1 1 1
  spline S249 degree 2 poles (-0.0267, 13.8542) (-0.0267, 13.7487) (-0.1201, 13.7487) knots 0 0 0 1 1 1
  spline S250 degree 2 poles (-0.1201, 13.7487) (-0.2136, 13.7487) (-0.352, 13.8542) knots 0 0 0 1 1 1
  spline S251 degree 2 poles (-0.352, 13.8542) (-0.4385, 13.9199) (-0.5682, 14.048) knots 0 0 0 1 1 1
  spline S252 degree 2 poles (-0.5682, 14.048) (-0.672, 14.1535) (-0.6824, 14.1535) knots 0 0 0 1 1 1
  spline S253 degree 2 poles (-0.6824, 14.1535) (-0.7032, 14.1535) (-0.7032, 14.1293) knots 0 0 0 1 1 1
  spline S254 degree 2 poles (-0.7032, 14.1293) (-0.7032, 14.1085) (-0.6703, 13.9891) (-0.6599, 13.977) knots 0 0 0 1 2 2 2
  spline S255 degree 2 poles (-0.6599, 13.977) (-0.0302, 13.3144) (-0.0302, 13.0843) knots 0 0 0 1 1 1
  spline S256 degree 2 poles (-0.0302, 13.0843) (-0.0302, 13.067) (-0.0492, 13.067) knots 0 0 0 1 1 1
  spline S257 degree 2 poles (-0.0492, 13.067) (-0.0752, 13.067) (-0.0821, 13.1051) knots 0 0 0 1 1 1
  spline S258 degree 2 poles (-0.0821, 13.1051) (-0.0907, 13.1518) (-0.1271, 13.2296) knots 0 0 0 1 1 1
  spline S259 degree 2 poles (-0.1271, 13.2296) (-0.1772, 13.3455) (-0.3693, 13.5739) knots 0 0 0 1 1 1
  spline S260 degree 2 poles (-0.3693, 13.5739) (-0.5388, 13.7781) (-0.6617, 13.8888) knots 0 0 0 1 1 1
  line L56 (-0.6686, 14.8525) -> (-0.2914, 14.3975)
  spline S261 degree 2 poles (-0.2914, 14.3975) (-0.0302, 14.0532) (-0.0302, 13.9148) knots 0 0 0 1 1 1
  spline S262 degree 2 poles (-0.0302, 13.9148) (-0.0302, 13.8975) (-0.0492, 13.8975) knots 0 0 0 1 1 1
  spline S263 degree 2 poles (-0.0492, 13.8975) (-0.0752, 13.8975) (-0.0821, 13.9269) knots 0 0 0 1 1 1
  spline S264 degree 2 poles (-0.0821, 13.9269) (-0.108, 14.0307) (-0.1392, 14.0878) knots 0 0 0 1 1 1
  spline S265 degree 2 poles (-0.1392, 14.0878) (-0.1859, 14.1777) (-0.4143, 14.4649) knots 0 0 0 1 1 1
  spline S266 degree 2 poles (-0.4143, 14.4649) (-0.5146, 14.5947) (-0.7361, 14.8386) knots 0 0 0 1 1 1
  spline S267 degree 2 poles (-0.7361, 14.8386) (-0.8312, 14.9303) (-0.8312, 14.9701) knots 0 0 0 1 1 1
  spline S268 degree 2 poles (-0.8312, 14.9701) (-0.8312, 15.0497) (-0.7793, 15.0497) knots 0 0 0 1 1 1
  spline S269 degree 2 poles (-0.7793, 15.0497) (-0.7136, 15.0497) (-0.5077, 14.8888) knots 0 0 0 1 1 1
  spline S270 degree 2 poles (-0.5077, 14.8888) (-0.7932, 15.2002) (-0.7932, 15.3179) knots 0 0 0 1 1 1
  spline S271 degree 2 poles (-0.7932, 15.3179) (-0.7932, 15.3577) (-0.743, 15.4234) (-0.7049, 15.4234) knots 0 0 0 1 2 2 2
  spline S272 degree 2 poles (-0.7049, 15.4234) (-0.6478, 15.4234) (-0.5371, 15.3455) knots 0 0 0 1 1 1
  spline S273 degree 2 poles (-0.5371, 15.3455) (-0.8226, 15.6345) (-0.8226, 15.8006) knots 0 0 0 1 1 1
  spline S274 degree 2 poles (-0.8226, 15.8006) (-0.8226, 15.8957) (-0.7447, 15.8957) knots 0 0 0 1 1 1
  spline S275 degree 2 poles (-0.7447, 15.8957) (-0.6444, 15.8957) (-0.1634, 15.4269) (-0.115, 15.4269) knots 0 0 0 1 2 2 2
  spline S276 degree 2 poles (-0.115, 15.4269) (-0.0786, 15.4269) (-0.0769, 15.5272) (-0.0544, 15.5272) knots 0 0 0 1 2 2 2
  spline S277 degree 2 poles (-0.0544, 15.5272) (-0.0267, 15.5272) (-0.0267, 15.4442) knots 0 0 0 1 1 1
  spline S278 degree 2 poles (-0.0267, 15.4442) (-0.0267, 15.3317) (-0.1253, 15.3317) knots 0 0 0 1 1 1
  spline S279 degree 2 poles (-0.1253, 15.3317) (-0.2361, 15.3317) (-0.6997, 15.74) (-0.7274, 15.74) knots 0 0 0 1 2 2 2
  spline S280 degree 2 poles (-0.7274, 15.74) (-0.7447, 15.74) (-0.7447, 15.7193) knots 0 0 0 1 1 1
  spline S281 degree 2 poles (-0.7447, 15.7193) (-0.7447, 15.6327) (-0.4748, 15.3455) knots 0 0 0 1 1 1
  spline S282 degree 2 poles (-0.4748, 15.3455) (-0.2516, 15.1068) (-0.1132, 14.9943) knots 0 0 0 1 1 1
  spline S283 degree 2 poles (-0.1132, 14.9943) (-0.0267, 14.9251) (-0.0267, 14.8923) knots 0 0 0 1 1 1
  spline S284 degree 2 poles (-0.0267, 14.8923) (-0.0267, 14.8369) (-0.0786, 14.8369) knots 0 0 0 1 1 1
  spline S285 degree 2 poles (-0.0786, 14.8369) (-0.1305, 14.8369) (-0.6305, 15.285) (-0.6893, 15.285) knots 0 0 0 1 2 2 2
  spline S286 degree 2 poles (-0.6893, 15.285) (-0.7153, 15.285) (-0.7153, 15.2573) knots 0 0 0 1 1 1
  spline S287 degree 2 poles (-0.7153, 15.2573) (-0.7153, 15.1829) (-0.4662, 14.9182) knots 0 0 0 1 1 1
  spline S288 degree 2 poles (-0.4662, 14.9182) (-0.2534, 14.6916) (-0.1323, 14.5981) knots 0 0 0 1 1 1
  spline S289 degree 2 poles (-0.1323, 14.5981) (-0.0388, 14.5255) (-0.0388, 14.4718) knots 0 0 0 1 1 1
  spline S290 degree 2 poles (-0.0388, 14.4718) (-0.0388, 14.4234) (-0.0821, 14.4234) knots 0 0 0 1 1 1
  spline S291 degree 2 poles (-0.0821, 14.4234) (-0.1357, 14.4234) (-0.3831, 14.6224) knots 0 0 0 1 1 1
  line L57 (-0.3831, 14.6224) -> (-0.6686, 14.8525)
  spline S292 degree 2 poles (-0.3312, 16.0307) (-0.0302, 15.6483) (-0.0302, 15.5047) knots 0 0 0 1 1 1
  spline S293 degree 2 poles (-0.0302, 15.5047) (-0.0302, 15.4874) (-0.0492, 15.4874) knots 0 0 0 1 1 1
  spline S294 degree 2 poles (-0.0492, 15.4874) (-0.0769, 15.4874) (-0.0821, 15.522) knots 0 0 0 1 1 1
  spline S295 degree 2 poles (-0.0821, 15.522) (-0.1028, 15.6552) (-0.2897, 15.894) knots 0 0 0 1 1 1
  line L58 (-0.2897, 15.894) -> (-0.4333, 16.0774)
  line L59 (-0.4333, 16.0774) -> (-0.6686, 16.3732)
  spline S296 degree 2 poles (-0.6686, 16.3732) (-0.8087, 16.5757) (-0.8087, 16.721) knots 0 0 0 1 1 1
  spline S297 degree 2 poles (-0.8087, 16.721) (-0.8087, 16.8282) (-0.7015, 16.8404) knots 0 0 0 1 1 1
  spline S298 degree 2 poles (-0.7015, 16.8404) (-0.7551, 16.8957) (-0.7551, 16.9182) knots 0 0 0 1 1 1
  spline S299 degree 2 poles (-0.7551, 16.9182) (-0.7551, 16.9649) (-0.7153, 16.9649) knots 0 0 0 1 1 1
  spline S300 degree 2 poles (-0.7153, 16.9649) (-0.6651, 16.9649) (-0.1547, 16.5272) (-0.1115, 16.5272) knots 0 0 0 1 2 2 2
  spline S301 degree 2 poles (-0.1115, 16.5272) (-0.0821, 16.5272) (-0.0786, 16.6189) (-0.0561, 16.6189) knots 0 0 0 1 2 2 2
  spline S302 degree 2 poles (-0.0561, 16.6189) (-0.0267, 16.6189) (-0.0267, 16.5238) knots 0 0 0 1 1 1
  spline S303 degree 2 poles (-0.0267, 16.5238) (-0.0267, 16.4286) (-0.1115, 16.4286) knots 0 0 0 1 1 1
  spline S304 degree 2 poles (-0.1115, 16.4286) (-0.179, 16.4286) (-0.3018, 16.5047) knots 0 0 0 1 1 1
  line L60 (-0.3018, 16.5047) -> (-0.1513, 16.3282)
  spline S305 degree 2 poles (-0.1513, 16.3282) (-0.0544, 16.1985) (-0.0544, 16.1206) knots 0 0 0 1 1 1
  spline S306 degree 2 poles (-0.0544, 16.1206) (-0.0544, 15.9978) (-0.179, 15.9978) knots 0 0 0 1 1 1
  spline S307 degree 2 poles (-0.179, 15.9978) (-0.2482, 15.9978) (-0.3312, 16.0307) knots 0 0 0 1 1 1
  spline S308 degree 2 poles (-0.7499, 16.74) (-0.7499, 16.6552) (-0.2464, 16.1276) (-0.1617, 16.1276) knots 0 0 0 1 2 2 2
  spline S309 degree 2 poles (-0.1617, 16.1276) (-0.1236, 16.1276) (-0.1236, 16.1639) knots 0 0 0 1 1 1
  spline S310 degree 2 poles (-0.1236, 16.1639) (-0.1236, 16.2469) (-0.6167, 16.7815) (-0.7032, 16.7815) knots 0 0 0 1 2 2 2
  spline S311 degree 2 poles (-0.7032, 16.7815) (-0.7499, 16.7815) (-0.7499, 16.74) knots 0 0 0 1 1 1
  spline S312 degree 2 poles (-0.4627, 17.548) (-0.7949, 17.9407) (-0.7949, 18.0981) knots 0 0 0 1 1 1
  spline S313 degree 2 poles (-0.7949, 18.0981) (-0.7949, 18.2002) (-0.6997, 18.2002) knots 0 0 0 1 1 1
  spline S314 degree 2 poles (-0.6997, 18.2002) (-0.615, 18.2002) (-0.1738, 17.7417) (-0.1288, 17.7417) knots 0 0 0 1 2 2 2
  spline S315 degree 2 poles (-0.1288, 17.7417) (-0.0821, 17.7417) (-0.0752, 17.8455) (-0.0544, 17.8455) knots 0 0 0 1 2 2 2
  spline S316 degree 2 poles (-0.0544, 17.8455) (-0.0267, 17.8455) (-0.0267, 17.7417) knots 0 0 0 1 1 1
  spline S317 degree 2 poles (-0.0267, 17.7417) (-0.0267, 17.6224) (-0.1323, 17.6224) knots 0 0 0 1 1 1
  spline S318 degree 2 poles (-0.1323, 17.6224) (-0.2205, 17.6224) (-0.3572, 17.7366) knots 0 0 0 1 1 1
  spline S319 degree 2 poles (-0.3572, 17.7366) (-0.4264, 17.7954) (-0.5717, 17.9476) knots 0 0 0 1 1 1
  spline S320 degree 2 poles (-0.5717, 17.9476) (-0.6807, 18.0618) (-0.7032, 18.0618) knots 0 0 0 1 1 1
  spline S321 degree 2 poles (-0.7032, 18.0618) (-0.7222, 18.0618) (-0.7222, 18.0359) knots 0 0 0 1 1 1
  spline S322 degree 2 poles (-0.7222, 18.0359) (-0.7222, 17.9545) (-0.5042, 17.6829) knots 0 0 0 1 1 1
  spline S323 degree 2 poles (-0.5042, 17.6829) (-0.3243, 17.4545) (-0.2084, 17.3455) knots 0 0 0 1 1 1
  spline S324 degree 2 poles (-0.2084, 17.3455) (-0.0613, 17.2054) (-0.0613, 17.176) knots 0 0 0 1 1 1
  spline S325 degree 2 poles (-0.0613, 17.176) (-0.0613, 17.1518) (-0.1063, 17.1154) (-0.1305, 17.1154) knots 0 0 0 1 2 2 2
  spline S326 degree 2 poles (-0.1305, 17.1154) (-0.1634, 17.1154) (-0.3952, 17.3127) knots 0 0 0 1 1 1
  line L61 (-0.3952, 17.3127) -> (-0.672, 17.548)
  line L62 (-0.672, 17.548) -> (-0.3762, 17.1829)
  line L63 (-0.3762, 17.1829) -> (-0.1703, 16.913)
  spline S327 degree 2 poles (-0.1703, 16.913) (-0.0302, 16.7071) (-0.0302, 16.5981) knots 0 0 0 1 1 1
  spline S328 degree 2 poles (-0.0302, 16.5981) (-0.0302, 16.5791) (-0.0475, 16.5791) knots 0 0 0 1 1 1
  spline S329 degree 2 poles (-0.0475, 16.5791) (-0.0734, 16.5791) (-0.0821, 16.6189) knots 0 0 0 1 1 1
  spline S330 degree 2 poles (-0.0821, 16.6189) (-0.0925, 16.6725) (-0.1253, 16.7469) knots 0 0 0 1 1 1
  spline S331 degree 2 poles (-0.1253, 16.7469) (-0.1703, 16.8507) (-0.4298, 17.1708) knots 0 0 0 1 1 1
  spline S332 degree 2 poles (-0.4298, 17.1708) (-0.6634, 17.4597) (-0.7862, 17.586) knots 0 0 0 1 1 1
  spline S333 degree 2 poles (-0.7862, 17.586) (-0.8087, 17.6085) (-0.8381, 17.6535) knots 0 0 0 1 1 1
  spline S334 degree 2 poles (-0.8381, 17.6535) (-0.8468, 17.676) (-0.8468, 17.702) knots 0 0 0 1 1 1
  spline S335 degree 2 poles (-0.8468, 17.702) (-0.8468, 17.7262) (-0.8139, 17.7763) (-0.7914, 17.7763) knots 0 0 0 1 2 2 2
  spline S336 degree 2 poles (-0.7914, 17.7763) (-0.7655, 17.7763) (-0.4627, 17.548) knots 0 0 0 1 1 1
  point P0 (1, 0)
  constraints: 2 other
emboss "Emboss1" sketch "Sketch8" operation cut depth 1 direction (-1, 0, 0)
body "Solid1"
